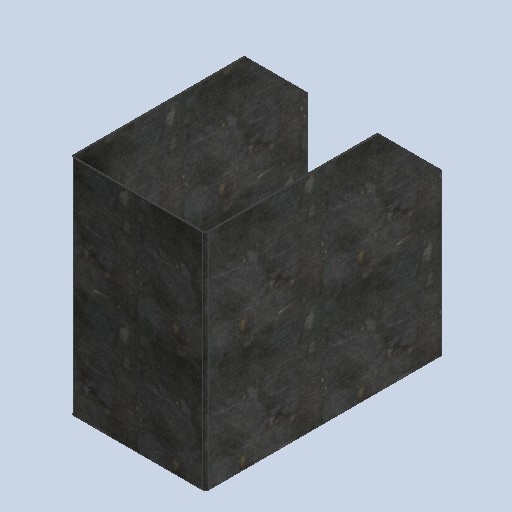
# Autodesk Inventor part: LzC-StoveCover
Saved by Autodesk Inventor 2024.3 (Build 283343000, 343)
## iProperties
Created: 2025-06-17
Part Number: LzC-StoveCover
Material: Steel
Document SubType Name: Sheet Metal
Designer: ajclo
Density: 7.85 g/cm^3
Sheet Metal Rule: Default_mm
Appearance: Plate
Flat Pattern Width: 33.178 cm
Flat Pattern Length: 89.3048 cm
Flat Pattern Area: 2962.95 cm^2
Sheet Metal Width: 331,780 mm
Sheet Metal Length: 893,048 mm
Sheet Metal Area: 296295,395 mm^2
Mass: 4519.41 g
Surface Area: 5804.05 cm^2
Volume: 575.721 cm^3
Author: ajclo
Autodesk Inventor part; units mm, degrees
ref_plane "YZ Plane" through (0, 0, 0) normal (1, 0, 0) x (0, 1, 0)
ref_plane "XZ Plane" through (0, 0, 0) normal (0, 1, 0) x (-1, 0, 0)
ref_plane "XY Plane" through (0, 0, 0) normal (0, 0, 1) x (1, 0, 0)
sketch "Sketch1" plane through (0, 0, 0) normal (1, 0, 0) x (0, 1, 0)
  line L0 (0, 0) -> (331.78, 0)
  line L1 (331.78, 0) -> (331.78, -350)
  line L2 (331.78, -350) -> (0, -350)
  line L3 (0, -350) -> (0, 0)
  line L4 (239.261, -350) -> (331.78, -257.481)
  line L5 (120, -350) -> (115, -350)
  line L6 (115, -350) -> (115, -353)
  line L7 (115, -353) -> (120, -353)
  line L8 (120, -353) -> (120, -350)
  line L9 (115, -353) -> (130, -353)
  line L10 (130, -353) -> (130, -358)
  line L11 (130, -358) -> (115, -358)
  line L12 (115, -358) -> (115, -353)
  line L13 (90, -350) -> (95, -350)
  line L14 (95, -350) -> (95, -353)
  line L15 (95, -353) -> (90, -353)
  line L16 (90, -353) -> (90, -350)
  line L17 (90, -353) -> (105, -353)
  line L18 (105, -353) -> (105, -358)
  line L19 (105, -358) -> (90, -358)
  line L20 (90, -358) -> (90, -353)
  line L21 (60, -350) -> (65, -350)
  line L22 (65, -350) -> (65, -353)
  line L23 (65, -353) -> (60, -353)
  line L24 (60, -353) -> (60, -350)
  line L25 (60, -353) -> (75, -353)
  line L26 (75, -353) -> (75, -358)
  line L27 (75, -358) -> (60, -358)
  line L28 (60, -358) -> (60, -353)
  point P0 (117.5, -353)
  point P1 (115, -355.5)
  point P2 (130, -355.5)
  point P3 (95, -351.5)
  point P4 (90, -351.5)
  point P5 (90, -355.5)
  point P6 (60, -351.5)
  point P7 (65, -351.5)
  dimension "d0" = 350
  dimension "d1" = 331.78
  dimension "d2" = 239.261
  dimension "d3" = 45
  dimension "d27" = 3
  dimension "d28" = 5
  dimension "d29" = 5
  dimension "d30" = 15
  dimension "d31" = 115
  dimension "d32" = 5
  dimension "d33" = 15
  dimension "d34" = 5
  dimension "d35" = 25
  dimension "d36" = 15
  dimension "d37" = 5
  dimension "d38" = 65
  measures "d0" distance of L2.end L0.start
  measures "d1" distance of L1.end L2.end
  measures "d2" distance of L2.end L4.start
  measures "d3" angle of L2 L4
  measures "d27" distance of L7.end L5.start
  measures "d28" distance between parallel lines of L8 L6
  measures "d29" distance from line of L11 point (117.5, -353)
  measures "d30" distance of point (115, -355.5) point (130, -355.5)
  measures "d31" distance between parallel lines of L3 L6
  measures "d32" distance of L17.end L18.end
  measures "d33" distance of L18.end L19.end
  measures "d34" distance of point (95, -351.5) point (90, -351.5)
  measures "d35" distance of point (115, -355.5) point (90, -355.5)
  measures "d36" distance of L26.end L27.end
  measures "d37" distance of point (60, -351.5) point (65, -351.5)
  measures "d38" distance from line of L3 point (65, -351.5)
extrude "Plate1" add sketch "Sketch1" along normal blind 2 contours L0 L1 L4 L2 L3 | L2 L22 L23 L24 | L23 L25 L26 L27 L28 | L8 L7 L6 L2 | L2 L14 L15 L16 | L9 L10 L11 L12 L7 | L15 L17 L18 L19 L20
sketch "Sketch2" plane through (0, 0, -2) normal (0, 0, 1) x (1, 0, 0)
  line L0 (0, 331.78) -> (0, 0)
  line L1 (0, 0) -> (200, 0)
  line L2 (200, 0) -> (200, 331.78)
  line L3 (200, 331.78) -> (0, 331.78)
  constraints: 6 end point, 1 horizontal, 1 perpendicular, 1 vertical
edge flange "Flange1" height 200 angle 90 thickness 2 bend radius 2 thickness toward (0, 0, 1) relief tear relief width 2 relief depth 1 edges at (2, 165.89, 0) wall of the first edge with corners at (0, 331.78, -2) (0, 0, -2) (200, 0, -2) (200, 331.78, -2)
bend "Bend1"
corner "Corner1"
sketch "Sketch3" plane through (198, 0, 0) normal (1, 0, 0) x (0, 1, 0)
  line L0 (331.78, 0) -> (0, 0)
  line L1 (0, 0) -> (0, -350)
  line L2 (0, -350) -> (331.78, -350)
  line L3 (331.78, -350) -> (331.78, 0)
  constraints: 6 end point, 1 horizontal, 1 perpendicular, 1 vertical
edge flange "Flange2" height 350 angle 90 thickness 2 bend radius 2 thickness toward (1, 0, 0) relief tear relief width 2 relief depth 1 edges at (200, 165.89, -2) wall of the first edge with corners at (198, 331.78, 0) (198, 0, 0) (198, 0, -350) (198, 331.78, -350)
bend "Bend2"
corner "Corner2"
sketch "Sketch4" plane through (200, 0, -350) normal (1, 0, 0) x (0, 0, -1)
  line L0 (-92.519, 331.78) -> (0, 239.261) projected
  line L1 (-346, 331.78) -> (0, 331.78) projected
  line L2 (0, 331.78) -> (0, 0) projected
  point P0 (-350, 0)
extrude "Cut1" cut sketch "Sketch4" against normal blind 2
sketch "Sketch5" plane through (200, 0, -4) normal (1, 0, 0) x (0, 0, -1)
  line L0 (0, 331.78) -> (0, 0)
  line L1 (346, 0) -> (0, 0)
  line L2 (346, 60) -> (346, 0)
  line L3 (354, 60) -> (346, 60)
  line L4 (354, 75) -> (354, 60)
  line L5 (349, 75) -> (354, 75)
  line L6 (349, 65) -> (349, 75)
  line L7 (346, 65) -> (349, 65)
  line L8 (346, 90) -> (346, 65)
  line L9 (354, 90) -> (346, 90)
  line L10 (354, 105) -> (354, 90)
  line L11 (349, 105) -> (354, 105)
  line L12 (349, 95) -> (349, 105)
  line L13 (346, 95) -> (349, 95)
  line L14 (346, 115) -> (346, 95)
  line L15 (354, 115) -> (346, 115)
  line L16 (354, 130) -> (354, 115)
  line L17 (349, 130) -> (354, 130)
  line L18 (349, 120) -> (349, 130)
  line L19 (346, 120) -> (349, 120)
  line L20 (346, 239.261) -> (346, 120)
  line L21 (253.481, 331.78) -> (346, 239.261)
  line L22 (0, 331.78) -> (253.481, 331.78)
  line L23 (346, 239.261) -> (253.481, 331.78)
  line L24 (0, 331.78) -> (253.481, 331.78)
  line L25 (0, 331.78) -> (0, 0)
  line L26 (346, 0) -> (0, 0)
  line L27 (346, 239.261) -> (346, 0)
  line L28 (346, 120) -> (354, 120)
  line L29 (354, 120) -> (354, 115)
  line L30 (354, 115) -> (346, 115)
  line L31 (346, 115) -> (346, 120)
  line L32 (354, 90) -> (346, 90)
  line L33 (346, 95) -> (354, 95)
  line L34 (354, 95) -> (354, 90)
  line L35 (354, 90) -> (346, 90)
  line L36 (346, 90) -> (346, 95)
  line L37 (346, 65) -> (354, 65)
  line L38 (354, 65) -> (354, 60)
  line L39 (354, 60) -> (346, 60)
  line L40 (346, 60) -> (346, 65)
  line L41 (354, 65) -> (349, 65)
  line L42 (349, 65) -> (349, 75)
  line L43 (349, 75) -> (354, 75)
  line L44 (354, 75) -> (354, 65)
  line L45 (354, 95) -> (349, 95)
  line L46 (349, 95) -> (349, 105)
  line L47 (349, 105) -> (354, 105)
  line L48 (354, 105) -> (354, 95)
  line L49 (354, 120) -> (349, 120)
  line L50 (349, 120) -> (349, 130)
  line L51 (349, 130) -> (354, 130)
  line L52 (354, 130) -> (354, 120)
  point P0 (-4, 0)
  point P1 (346, 65)
  point P2 (346, 60)
  point P3 (346, 95)
  point P4 (346, 90)
  point P5 (346, 120)
  point P6 (346, 115)
sheet face with bend "Face2" sketch "Sketch5" thickness 2 toward (-1, 0, 0) bend radius 2 contours L27 L7 L37 L4 L3 | L19 L28 L16 L15 L27 | L18 L17 L16 L28 | L37 L6 L5 L4 | L27 L13 L33 L10 L9 | L12 L11 L10 L33
bend "Bend3"
sketch "Sketch6" plane through (0, 0, 0) normal (-1, 0, 0) x (0, 0, 1)
  line L0 (-4, 0) -> (-4, 331.78) projected
  line L1 (-257.481, 331.78) -> (-4, 331.78) projected
  line L2 (-350, 239.261) -> (-257.481, 331.78) projected
  line L3 (-350, 120) -> (-350, 239.261) projected
  line L4 (-353, 120) -> (-350, 120) projected
  line L5 (-353, 130) -> (-353, 120) projected
  line L6 (-358, 130) -> (-353, 130) projected
  line L7 (-358, 115) -> (-358, 130) projected
  line L8 (-350, 115) -> (-358, 115) projected
  line L9 (-350, 95) -> (-350, 115) projected
  line L10 (-353, 95) -> (-350, 95) projected
  line L11 (-353, 105) -> (-353, 95) projected
  line L12 (-358, 105) -> (-353, 105) projected
  line L13 (-358, 90) -> (-358, 105) projected
  line L14 (-350, 90) -> (-358, 90) projected
  line L15 (-350, 65) -> (-350, 90) projected
  line L16 (-353, 65) -> (-350, 65) projected
  line L17 (-353, 75) -> (-353, 65) projected
  line L18 (-358, 75) -> (-353, 75) projected
  line L19 (-358, 60) -> (-358, 75) projected
  line L20 (-350, 60) -> (-358, 60) projected
  line L21 (-350, 0) -> (-350, 60) projected
  line L22 (-4, 0) -> (-350, 0) projected
  line L23 (-350, 60) -> (-350, 120)
  line L24 (-350, 120) -> (-353, 120)
  line L25 (-353, 130) -> (-358, 130)
  line L26 (-358, 60) -> (-350, 60)
  line L27 (-358, 60) -> (-358, 130)
  point P0 (0, 0)
  constraints: 10 end point, 2 perpendicular, 1 collinear, 1 horizontal, 1 vertical
extrude "Extrusion1" cut sketch "Sketch6" against normal through all contours L20 L19 L18 L17 L16 L23 | L23 L8 L7 L6 L5 L4 | L14 L13 L12 L11 L10 L23
equation "\"d33\" = d30"
equation "\"d34\" = d28"
equation "\"d36\" = d33"
equation "\"d25\" = Thickness"
equation "\"d4\" = Thickness"
equation "\"d5\" = BendReliefWidth"
equation "\"d6\" = BendReliefDepth"
equation "\"d7\" = MinimumRemnant"
equation "\"d8\" = TransitionRadius"
equation "\"d11\" = BendRadius"
equation "\"d12\" = CornerReliefSize"
equation "\"d13\" = GapSize"
equation "\"d14\" = JacobiRadiusSize"
equation "\"d15\" = BendReliefWidth"
equation "\"d16\" = BendReliefDepth"
equation "\"d17\" = MinimumRemnant"
equation "\"d18\" = TransitionRadius"
equation "\"d21\" = BendRadius"
equation "\"d22\" = CornerReliefSize"
equation "\"d23\" = GapSize"
equation "\"d24\" = JacobiRadiusSize"
equation "\"d39\" = BendRadius"
equation "\"d40\" = BendReliefWidth"
equation "\"d42\" = MinimumRemnant"
equation "\"d41\" = BendReliefDepth"
equation "\"d43\" = TransitionRadius"
equation "\"d37\" = d34"
equation "\"BendRadius\" = Thickness"
equation "\"BendReliefWidth\" = Thickness"
equation "\"BendReliefDepth\" = 0.5 * Thickness"
equation "\"CornerReliefSize\" = 4 * Thickness"
equation "\"MinimumRemnant\" = 2 * Thickness"
equation "\"TransitionRadius\" = BendRadius"
equation "\"JacobiRadiusSize\" = BendRadius"
equation "\"GapSize\" = Thickness"
equation "\"Thickness\" = 2"
body "Solid1"
